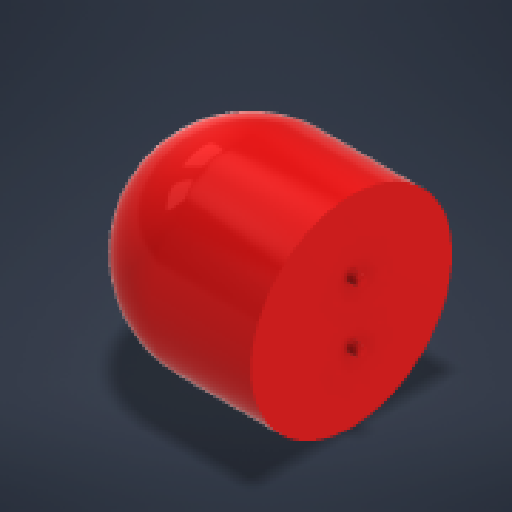
# Autodesk Inventor part: diffuser
Saved by Autodesk Inventor 2023 (Build 270158000, 158)
## iProperties
Created: 2023-12-07
Part Number: diffuser
Material: Generic
Document SubType Name: Modeling
Designer: Andi
Density: 1 g/cm^3
Appearance: Chestnut
Author: Andi
Autodesk Inventor part; units mm, degrees
ref_plane "YZ Plane" through (0, 0, 0) normal (1, 0, 0) x (0, 1, 0)
ref_plane "XZ Plane" through (0, 0, 0) normal (0, 1, 0) x (-1, 0, 0)
ref_plane "XY Plane" through (0, 0, 0) normal (0, 0, 1) x (1, 0, 0)
sketch "Sketch1" plane through (0, 0, 0) normal (0, 0, 1) x (1, 0, 0)
  line L0 (-5, 0) -> (5, 0)
  line L1 (0, -5) -> (5, -5) construction
  line L2 (5, 5) -> (0, 5)
  arc A0 (0, 5) -> (-5, 0) centre (0, 0) ccw
  line L3 (5, 5) -> (5, 0)
  arc A1 (-5, 0) -> (0, -5) centre (0, 0) ccw construction
  line L4 (5, 0) -> (5, -5) construction
  dimension "d0" = 10
  dimension "d1" = 5
  constraints: 12 end point, 4 point on circle, 4 tangent, 2 centre point, 2 coincident, 2 midpoint, 2 parallel, 2 vertical, 1 horizontal
  measures "d0" distance of L2.start L1.end
  measures "d1" distance from line of point (0, 0) L3
revolve "Revolution1" add sketch "Sketch1" angle 360 about axis through (-5, 0, 0) along (1, 0, 0)
sketch "Sketch2" plane through (5, 0, 0) normal (1, 0, 0) x (0, 0, -1)
  circle A0 centre (0, 1.5) radius 0.25
  circle A1 centre (0, -1.5) radius 0.25
  line L0 (0, 1.5) -> (0, -1.5) construction
  point P0 (0, 0)
  point P1 (0, 0)
  dimension "d3" = 3
  dimension "d4" = 0.5
  constraints: 2 centre point, 2 end point, 1 coincident, 1 equal radius, 1 midpoint, 1 vertical, 1 vertical alignment
  measures "d3" distance of L0.start L0.end
  measures "d4" diameter of A1
extrude "Extrusion1" add sketch "Sketch2" along normal blind 0.5
body "Solid1"
